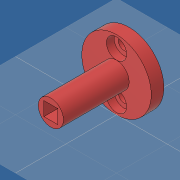
# Autodesk Inventor part: Schalter_Basis
Saved by Autodesk Inventor 2019 (Build 230136000, 136)
## iProperties
Created: 2020-08-07
Part Number: Schalter_Basis
Material: Generisch
Document SubType Name: Modeling
Designer: Stefan
Mass: 3.85917 g
Surface Area: 31.5711 cm^2
Volume: 3.85917 cm^3
Density: 1 g/cm^3
Appearance: Glatt - Rot
Author: Stefan
Autodesk Inventor part; units mm, degrees
ref_plane "YZ Plane" through (0, 0, 0) normal (1, 0, 0) x (0, 1, 0)
ref_plane "XZ Plane" through (0, 0, 0) normal (0, 1, 0) x (-1, 0, 0)
ref_plane "XY Plane" through (0, 0, 0) normal (0, 0, 1) x (1, 0, 0)
sketch "Skizze1" plane through (0, 0, 0) normal (0, 0, 1) x (1, 0, 0)
  circle A0 centre (0, 0) radius 13.75
  circle A1 centre (0, 0) radius 5
  line L0 (2.75, 2.75) -> (-2.75, 2.75)
  line L1 (-2.75, 2.75) -> (-2.75, -2.75)
  line L2 (-2.75, -2.75) -> (2.75, -2.75)
  line L3 (2.75, -2.75) -> (2.75, 2.75)
  line L4 (2.75, 2.75) -> (-2.75, -2.75) construction
  line L5 (-2.75, 2.75) -> (2.75, -2.75) construction
  line L6 (0, 13.75) -> (0, -13.75) construction
  circle A2 centre (0, 9) radius 4
  circle A3 centre (0, 9) radius 2.25
  circle A4 centre (0, -9) radius 4
  circle A5 centre (0, -9) radius 2.25
  line L7 (-13.75, 0) -> (13.75, 0) construction
  circle A6 centre (0, 0) radius 2
  dimension "d0" = 27.5
  dimension "d1" = 10
  dimension "d25" = 5.5
  dimension "d28" = 8
  dimension "d29" = 18
  dimension "d30" = 4.5
  dimension "d43" = 4
  constraints: 16 end point, 7 centre point, 6 coincident, 6 midpoint, 4 point on circle, 2 equal radius, 2 horizontal, 2 parallel, 2 perpendicular, 2 point on line, 1 symmetric about line, 1 vertical
  measures "d0" diameter of A0
  measures "d1" diameter of A1
  measures "d25" distance of L2.end L1.end
  measures "d28" diameter of A2
  measures "d29" distance of A4.centre A2.centre
  measures "d30" diameter of A5
  measures "d43" diameter of A6
extrude "Extrusion1" add sketch "Skizze1" against normal blind 5 contours A0 | A1 | A4 | A2 | L3 L2 L1 L0
extrude "Extrusion8" cut sketch "Skizze1" against normal blind 3 contours A4 | A2
extrude "Extrusion9" add sketch "Skizze1" along normal blind 26 contours A1
extrude "Extrusion12" add sketch "Skizze1" along normal blind 3.5 contours L3 L2 L1 L0
